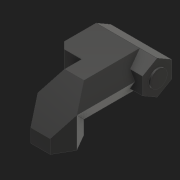
# Autodesk Inventor part: link_a0
Saved by Autodesk Inventor 2017 (Build 210142000, 142)
## iProperties
Created: 2019-08-03
Part Number: link_a0
Material: ABS Plastic
Document SubType Name: Modeling
Designer: Dell
Density: 1.06 g/cm^3
Appearance: Smooth - Black
Author: Dell
Autodesk Inventor part; units mm, degrees
ref_plane "YZ Plane" through (0, 0, 0) normal (1, 0, 0) x (0, 1, 0)
ref_plane "XZ Plane" through (0, 0, 0) normal (0, 1, 0) x (-1, 0, 0)
ref_plane "XY Plane" through (0, 0, 0) normal (0, 0, 1) x (1, 0, 0)
sketch "Sketch1" plane through (0, 0, 0) normal (0, 0, 1) x (1, 0, 0)
  line L0 (57.5, 0) -> (28.75, -49.7965)
  line L1 (28.75, -49.7965) -> (-28.75, -49.7965)
  line L2 (-28.75, -49.7965) -> (-57.5, 0)
  line L3 (-57.5, 0) -> (-28.75, 49.7965)
  line L4 (-28.75, 49.7965) -> (28.75, 49.7965)
  line L5 (28.75, 49.7965) -> (57.5, 0)
  point P0 (0, 0)
  point P1 (0, 0)
  dimension "d0" = 115
  constraints: 12 end point, 1 coincident, 13 other
  measures "d0" distance of L0.start L2.end
extrude "Extrusion1" add sketch "Sketch1" along normal blind 139.4929
sketch "Sketch2" plane through (-28.75, -49.7965, 0) normal (0, -1, 0) x (1, 0, 0)
  line L0 (-28.75, 89.6965) -> (0, 139.4929)
  line L1 (0, 139.4929) -> (57.5, 139.4929)
  line L2 (57.5, 139.4929) -> (86.25, 89.6965)
  line L3 (86.25, 89.6965) -> (57.5, 39.9)
  line L4 (57.5, 39.9) -> (0, 39.9)
  line L5 (0, 39.9) -> (-28.75, 89.6965)
  line L6 (0, 139.4929) -> (57.5, 139.4929) projected
  point P0 (28.75, 0)
  point P1 (28.75, 89.6965)
  point P2 (28.75, 139.4929)
  dimension "d3" = 115
  constraints: 12 end point, 2 midpoint, 1 point on line, 13 other
  measures "d3" distance of L2.end L0.start
extrude "Extrusion2" add sketch "Sketch2" against normal blind 307.5
sketch "Sketch3" plane through (0, 0, 139.4929) normal (0, 0, 1) x (1, 0, 0)
  line L0 (-28.75, 49.7965) -> (-28.75, 257.7035) projected
  line L1 (-28.75, 100.2035) -> (-100, 100.2035)
  line L2 (-100, 100.2035) -> (-100, 257.7035)
  line L3 (-57.5, 257.7035) -> (-28.75, 257.7035) projected
  line L4 (-100, 257.7035) -> (-28.75, 257.7035)
  line L5 (-80, 100.2035) -> (-100, 120.2035)
  point P0 (0, 0)
  dimension "d6" = 71.25
  dimension "d7" = 157.5
  dimension "d8" = 28.2843
  dimension "d9" = 45
  constraints: 8 end point, 3 point on line, 1 collinear, 1 horizontal, 1 perpendicular
  measures "d6" distance of L1.start L1.end
  measures "d7" distance of L1.end L2.end
  measures "d8" distance of L5.start L5.end
  measures "d9" angle of L1 L5
extrude "Extrusion3" add sketch "Sketch3" against normal blind 99.5929 contours L1 L5 L2 L4 L3 L0
sketch "Sketch4" plane through (-100, 120.2035, 139.4929) normal (-1, 0, 0) x (0, 0, 1)
  line L0 (-99.5929, 94.375) -> (-74.6947, 137.5)
  line L1 (-74.6947, 137.5) -> (-24.8982, 137.5)
  line L2 (-24.8982, 137.5) -> (0, 94.375)
  line L3 (0, 94.375) -> (-24.8982, 51.25)
  line L4 (-24.8982, 51.25) -> (-74.6947, 51.25)
  line L5 (-74.6947, 51.25) -> (-99.5929, 94.375)
  line L6 (0, 137.5) -> (-99.5929, 137.5) projected
  line L7 (0, 137.5) -> (0, 0) projected
  line L8 (-99.5929, 0) -> (-99.5929, 137.5) projected
  point P0 (-139.4929, -120.2035)
  point P1 (-49.7965, 94.375)
  point P2 (-49.7965, 137.5)
  constraints: 12 end point, 4 point on line, 1 midpoint, 1 vertical alignment, 13 other
extrude "Extrusion4" add sketch "Sketch4" against normal blind 180 contours L0 L1 L2 L3 L4 L5
sketch "Sketch6" plane through (80, 120.2035, 139.4929) normal (1, 0, 0) x (0, 0, -1)
  line L0 (0, 94.375) -> (24.8982, 137.5) projected
  line L1 (0, 137.5) -> (24.8982, 137.5) projected
  line L2 (0, 94.375) -> (0, 137.5) projected
  line L3 (74.6947, 137.5) -> (99.5929, 94.375) projected
  line L4 (99.5929, 94.375) -> (99.5929, 137.5) projected
  line L5 (74.6947, 137.5) -> (99.5929, 137.5) projected
  line L6 (49.7965, -120.2035) -> (99.5929, -170) projected
  line L7 (49.7965, -170) -> (49.7965, -120.2035) projected
  line L8 (99.5929, -170) -> (49.7965, -170) projected
  line L9 (0, -170) -> (49.7965, -120.2035) projected
  line L10 (49.7965, -170) -> (0, -170) projected
  line L11 (49.7965, -170) -> (49.7965, -120.2035) projected
  line L12 (0, -170) -> (49.7965, -120.2035) projected
  line L13 (49.7965, -120.2035) -> (0, -120.2035) projected
  line L14 (0, -170) -> (0, -120.2035) projected
  line L15 (49.7965, -120.2035) -> (0, -70.4071) projected
  line L16 (0, -120.2035) -> (0, -70.4071) projected
  line L17 (49.7965, -120.2035) -> (0, -120.2035) projected
  point P0 (139.4929, -120.2035)
extrude "Extrusion5" cut sketch "Sketch6" against normal through all
sketch "Sketch7" plane through (0, 0, 0) normal (0, 0, -1) x (-1, 0, 0)
  circle A0 centre (0, 0) radius 25
  dimension "d16" = 50
  constraints: 1 centre point, 1 coincident
  measures "d16" diameter of A0
extrude "Extrusion6" cut sketch "Sketch7" against normal blind 5
sketch "Sketch8" plane through (80, 120.2035, 139.4929) normal (1, 0, 0) x (0, 0, -1)
  line L0 (74.6947, 51.25) -> (99.5929, 94.375) projected
  line L1 (99.5929, 94.375) -> (74.6947, 137.5) projected
  line L2 (74.6947, 137.5) -> (24.8982, 137.5) projected
  line L3 (24.8982, 137.5) -> (0, 94.375) projected
  line L4 (0, 94.375) -> (24.8982, 51.25) projected
  line L5 (24.8982, 51.25) -> (74.6947, 51.25) projected
  circle A0 centre (49.7965, 94.375) radius 25
  point P0 (139.4929, -120.2035)
  point P1 (49.7965, 137.5)
  dimension "d19" = 50
  constraints: 1 centre point, 1 horizontal alignment, 1 midpoint, 1 vertical alignment
  measures "d19" diameter of A0
extrude "Extrusion7" add sketch "Sketch8" along normal blind 5 contours A0
body "Solid1"
